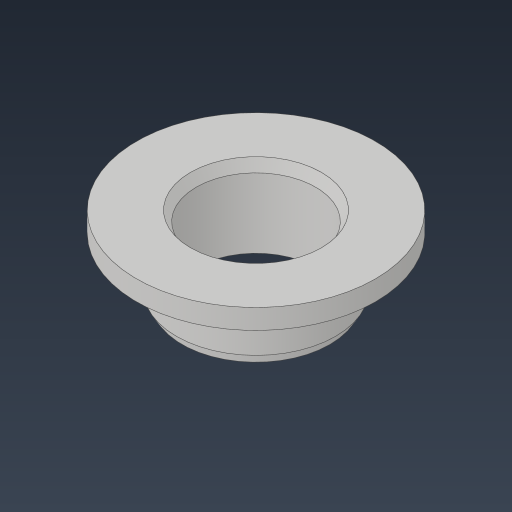
# Autodesk Inventor part: Lozysko GFM-0608-06
Saved by Autodesk Inventor 2023 (Build 270158000, 158)
## iProperties
Created: 2022-09-22
Part Number: Lozysko GFM-0608-06
Material: Ogólny
Document SubType Name: Modeling
Designer: Michał
Density: 1 g/cm^3
Appearance: Domyślna
Author: Michał
Autodesk Inventor part; units mm, degrees
ref_plane "YZ Plane" through (0, 0, 0) normal (1, 0, 0) x (0, 1, 0)
ref_plane "XZ Plane" through (0, 0, 0) normal (0, 1, 0) x (-1, 0, 0)
ref_plane "XY Plane" through (0, 0, 0) normal (0, 0, 1) x (1, 0, 0)
sketch "Szkic1" plane through (0, 0, 0) normal (0, 0, 1) x (1, 0, 0)
  line L0 (0, 0) -> (3, 0) construction
  line L1 (3, 0) -> (3, 3.5)
  line L2 (3, 3.5) -> (3.2887, 4)
  line L3 (3.2887, 4) -> (6, 4)
  line L4 (6, 4) -> (6, 3)
  line L5 (6, 3) -> (4, 3)
  line L6 (4, 3) -> (4, 0.5)
  line L7 (3.7113, 0) -> (3, 0)
  line L8 (3.7113, 0) -> (4, 0.5)
  line L9 (0, -0.8) -> (0, 4.8) projected
  dimension "d0" = 3
  dimension "d1" = 4
  dimension "d2" = 0.5
  dimension "d3" = 30
  dimension "d4" = 1
  dimension "d5" = 4
  dimension "d6" = 6
  constraints: 18 end point, 4 perpendicular, 3 parallel, 1 collinear, 1 horizontal, 1 point on line
  measures "d0" distance of L0.start L0.end
  measures "d1" distance from line of L0.start L6
  measures "d2" distance from line of L6.end L7
  measures "d3" angle of L6 L8
  measures "d4" distance between parallel lines of L3 L5
  measures "d5" distance between parallel lines of L7 L3
  measures "d6" distance from line of L0.start L4
revolve "Obrót1" add sketch "Szkic1" angle 360 about axis through (0, -10, 0) along (0, 1, 0)
